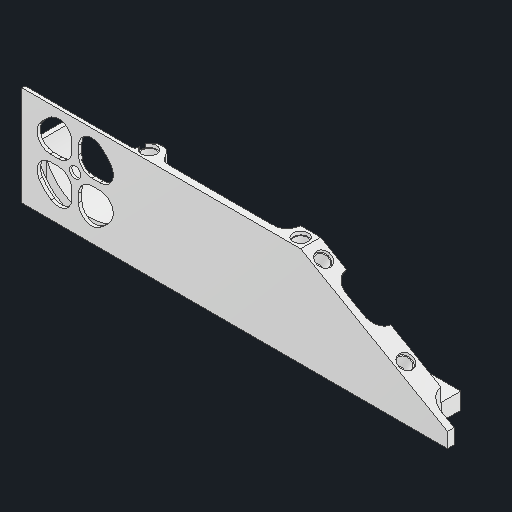
# Autodesk Inventor part: right_side
Saved by Autodesk Inventor 2023 (Build 270158000, 158)
## iProperties
Created: 2024-05-08
Part Number: right_side
Material: ABS Plastic
Document SubType Name: Modeling
Designer: szymo
Density: 1.06 g/cm^3
Appearance: Smooth - White
Mass: 9.52258 g
Surface Area: 89.3308 cm^2
Volume: 8.98357 cm^3
Author: szymo
Autodesk Inventor part; units mm, degrees
ref_plane "YZ Plane" through (0, 0, 0) normal (1, 0, 0) x (0, 1, 0)
ref_plane "XZ Plane" through (0, 0, 0) normal (0, 1, 0) x (-1, 0, 0)
ref_plane "XY Plane" through (0, 0, 0) normal (0, 0, 1) x (1, 0, 0)
sketch "Sketch1" plane through (0, 0, 0) normal (0, 0, 1) x (1, 0, 0)
  line L0 (128, 8) -> (128, 3.5) projected
  line L1 (128, 3.5) -> (132, 3.5) projected
  line L2 (132, 3.5) -> (132, 0) projected
  line L3 (132, 0) -> (146, 0) projected
  line L4 (146, 0) -> (132, 9) projected
  line L5 (132, 9) -> (132, 8) projected
  line L6 (132, 8) -> (128, 8) projected
  circle A0 centre (-25, 12) radius 22.5 projected
  line L7 (116.5, 3.5) -> (116.5, 11.1395) projected
  line L8 (116.5, 14.6395) -> (116.5, 11.1395) projected
  line L9 (109.1155, 18.903) -> (116.5, 14.6395)
  line L10 (109.1155, 18.903) -> (83.8327, 33.5)
  line L11 (47.75, 33.5) -> (83.8327, 33.5) projected
  line L12 (0, 3.5) -> (0, 31) projected
  line L13 (0, 3.5) -> (0, 33.5)
  line L14 (0, 33.5) -> (83.8327, 33.5)
  line L15 (83.8327, 33.5) -> (128, 8)
  line L16 (128, 3.5) -> (0, 3.5)
  point P0 (0, 0)
  constraints: 12 end point, 2 collinear, 1 parallel, 1 point on line
extrude "Extrusion1" add sketch "Sketch1" against normal blind 2 contours L0 L16 L7 L8 L15 | L8 L7 L16 L12 L13 L14 L11 L10 L9
sketch "Sketch2" plane through (0, 0, -2) normal (0, 0, -1) x (-1, 0, 0)
  circle A0 centre (-16, 19.5) radius 14 projected
  line L0 (0, 33.5) -> (-83.8327, 33.5) projected
  line L1 (-128, 3.5) -> (0, 3.5) projected
  line L2 (-33, 33.5) -> (0, 33.5)
  line L3 (0, 33.5) -> (0, 3.5)
  line L4 (0, 3.5) -> (-33, 3.5)
  line L5 (-33, 3.5) -> (-33, 33.5)
  point P0 (0, 0)
  point P1 (-116.5, 3.5)
  point P2 (-33, 3.5)
  dimension "d2" = 28
  dimension "d3" = 17
  constraints: 8 end point, 2 parallel, 1 horizontal, 1 perpendicular, 1 point on line
  measures "d2" diameter of A0
  measures "d3" distance from line of L5 A0.centre
extrude "Extrusion2" cut sketch "Sketch2" against normal blind 1 contours A0 | L0 L3 L1 L5
sketch "Sketch3" plane through (0, 0, -1) normal (0, 0, -1) x (-1, 0, 0)
  circle A0 centre (-16, 19.5) radius 14 projected
  line L0 (-33, 33.5) -> (0, 33.5) projected
  line L1 (-33, 3.5) -> (-33, 33.5) projected
  line L2 (0, 3.5) -> (-33, 3.5) projected
  line L3 (0, 33.5) -> (0, 3.5) projected
  line L4 (0, 3.5) -> (-128, 3.5) projected
  line L5 (0, 3.5) -> (-5, 3.5)
  line L6 (-5, 3.5) -> (-5, 6.5)
  line L7 (-5, 6.5) -> (0, 6.5)
  line L8 (0, 6.5) -> (0, 3.5)
  line L9 (-33, 3.5) -> (-28, 3.5)
  line L10 (-28, 3.5) -> (-28, 6.5)
  line L11 (-28, 6.5) -> (-33, 6.5)
  line L12 (-33, 6.5) -> (-33, 3.5)
  line L13 (-33, 9.5) -> (-25.798, 9.5)
  line L14 (-2.0052, 19.1168) -> (0, 18.5)
  line L15 (0, 33.5) -> (0, 3.5) projected
  point P0 (0, 0)
  point P1 (-116.5, 3.5)
  point P2 (0, 18.5)
  dimension "d6" = 5
  dimension "d7" = 3
  dimension "d8" = 5
  dimension "d9" = 3
  dimension "d10" = 3
  constraints: 20 end point, 4 parallel, 3 perpendicular, 3 point on line, 2 horizontal, 2 point on circle, 1 midpoint
  measures "d6" distance of L6.end L7.end
  measures "d7" distance of L5.end L6.end
  measures "d8" distance of L11.end L10.end
  measures "d9" distance of L10.end L9.end
  measures "d10" distance between parallel lines of L13 L11
ref_plane "Work Plane1" through (1, 4.5, -18.6) normal (0, 0, 1) x (1, 0, 0)
ref_plane "Work Plane2" through (1.675, 5.175, -4.8) normal (0, 0, 1) x (1, 0, 0)
extrude "Extrusion3" add sketch "Sketch3" along normal blind 6.8 contours A0 L14 L3 L7 L6 L2 L10 L11 L1 L13 | L11 L10 L2 L1 | L3 L2 L6 L7
sketch "Sketch4" plane through (0, 0, -7.8) normal (0, 0, -1) x (-1, 0, 0)
  circle A0 centre (-16, 19.5) radius 14 projected
  line L0 (-2.0052, 19.1168) -> (0, 18.5) projected
  line L1 (0, 33.5) -> (0, 18.5) projected
  line L2 (-33, 33.5) -> (0, 33.5) projected
  line L3 (-33, 9.5) -> (-33, 33.5) projected
  line L4 (-33, 9.5) -> (-25.798, 9.5) projected
  arc A1 (-25.798, 9.5) -> (-2.0052, 19.1168) centre (-16, 19.5) ccw projected
  line L5 (-29.9991, 19.6621) -> (-33, 19.6621)
  line L6 (-33, 9.5) -> (-33, 33.5) projected
  line L7 (0, 18.5) -> (-2.0052, 19.1168) projected
  line L8 (-2.0052, 19.1168) -> (0, 18.5)
  arc A2 (-25.798, 9.5) -> (-2.0052, 19.1168) centre (-16, 19.5) ccw projected
  line L9 (-25.798, 9.5) -> (-33, 9.5) projected
  line L10 (-33, 9.5) -> (-33, 3.5) projected
  line L11 (-33, 3.5) -> (0, 3.5) projected
  line L12 (0, 3.5) -> (0, 18.5) projected
  line L13 (0, 18.5) -> (-2.0052, 19.1168) projected
  point P0 (0, 0)
  constraints: 4 end point, 1 collinear, 1 perpendicular, 1 point on line, 2 other
ref_plane "Work Plane3" through (1, 4.5, -18.6) normal (0, 0, 1) x (1, 0, 0)
extrude "Extrusion4" add sketch "Sketch4" along normal blind 5 contours A0 L4 L3 L5 | A0 L0 L12 L11 L10 L4
sketch "Sketch5" plane through (25.798, 9.5, -1) normal (0, 1, 0) x (1, 0, 0)
  line L0 (7.202, 0) -> (0, 0) projected
  line L1 (7.202, 1) -> (7.202, 0) projected
  line L2 (7.202, 1) -> (7.202, 6.8) projected
  line L3 (0, 6.8) -> (7.202, 6.8) projected
  line L4 (0, 0) -> (0, 6.8) projected
  line L5 (7.202, 0) -> (0, 6.8)
  line L6 (0.7816, 0) -> (7.202, 6.8)
  point P0 (-25.798, -1)
  point P1 (3.9918, 3.4)
  constraints: 4 end point, 1 midpoint, 1 perpendicular, 1 point on line
hole "Hole1" at (29.7898, 9.5, -4.4) direction (0, -1, 0) diameter 3.6 end through all countersink diameter 6.5 countersink angle 90 clearance for "Countersunk Flat Head Screw ISO 2009/7046" size "M3" standard "ISO"
ref_plane "Work Plane4" through (41, 3.5, -89) normal (0, 1, 0) x (-1, 0, 0)
sketch "Sketch6" plane through (41, 3.5, -89) normal (0, 1, 0) x (-1, 0, 0)
  line L0 (8, 87) -> (-42.8327, 87) projected
  line L1 (-42.8327, 87) -> (-87, 87) projected
  line L2 (-87, 87) -> (8, 87) projected
  line L3 (-71, 89) -> (-71, 74) projected
  line L4 (-71, 74) -> (-87, 74) projected
  line L5 (-71, 87) -> (-64, 87)
  line L6 (-64, 87) -> (-64, 77)
  line L7 (-64, 77) -> (-71, 77)
  line L8 (-71, 77) -> (-71, 87)
  point P0 (41, 89)
  point P1 (-64, 87)
  dimension "d22" = 7
  dimension "d23" = 10
  constraints: 8 end point, 2 parallel, 2 point on line, 1 horizontal, 1 perpendicular
  measures "d22" distance of L6.end L7.end
  measures "d23" distance of L5.end L6.end
extrude "Extrusion5" add sketch "Sketch6" along normal blind 5
sketch "Sketch7" plane through (0, 0, -2) normal (0, 0, -1) x (-1, 0, 0)
  line L0 (-105, 8.5) -> (-105, 3.5) projected
  line L1 (-105, 3.5) -> (-33, 3.5) projected
  line L2 (-33, 3.5) -> (-33, 9.5) projected
  line L3 (-33, 9.5) -> (-33, 33.5) projected
  line L4 (-33, 33.5) -> (-83.8327, 33.5) projected
  line L5 (-83.8327, 33.5) -> (-128, 8) projected
  line L6 (-128, 8) -> (-128, 3.5) projected
  line L7 (-128, 3.5) -> (-112, 3.5) projected
  line L8 (-112, 3.5) -> (-112, 8.5) projected
  line L9 (-112, 8.5) -> (-105, 8.5) projected
  line L10 (-118.25, 3.5) -> (-115.75, 3.5) projected
  line L11 (-115.75, 3.5) -> (-118.25, 3.5)
  line L12 (-118.25, 3.5) -> (-118.25, 8.5)
  line L13 (-118.25, 8.5) -> (-115.75, 8.5)
  line L14 (-115.75, 8.5) -> (-115.75, 3.5)
  line L15 (-114, 3.5) -> (-120, 3.5)
  line L16 (-120, 3.5) -> (-120, 8.5)
  line L17 (-120, 8.5) -> (-114, 8.5)
  line L18 (-114, 8.5) -> (-114, 3.5)
  line L19 (-112, 8.5) -> (-114, 8.5)
  point P0 (0, 0)
  dimension "d26" = 5
  dimension "d27" = 6
  dimension "d28" = 1.75
  dimension "d29" = 1.75
  constraints: 18 end point, 4 parallel, 2 coincident, 2 horizontal, 2 perpendicular, 2 point on line, 1 collinear
  measures "d26" distance of L11.end L12.end
  measures "d27" distance of L16.end L17.end
  measures "d28" distance between parallel lines of L16 L12
  measures "d29" distance between parallel lines of L14 L18
extrude "Extrusion6" add sketch "Sketch7" along normal blind 10 contours L8 L7 L18 L19 | L18 L7 L14 L17 | L14 L7 L12 L13 | L12 L7 L16 L17
sketch "Sketch8" plane through (41, 8.5, -89) normal (0, 1, 0) x (1, 0, 0)
  line L0 (64, -77) -> (64, -87) projected
  line L1 (79, -87) -> (64, -87) projected
  line L2 (79, -87) -> (79, -77) projected
  line L3 (64, -77) -> (79, -77) projected
  line L4 (71, -77) -> (64, -83)
  line L5 (71, -89) -> (71, -74) projected
  point P0 (-41, -89)
  point P1 (67.5, -80)
  dimension "d40" = 4
  constraints: 3 point on line, 2 end point, 1 midpoint
  measures "d40" distance from line of L1 L4.end
hole "Hole2" at (108.5, 8.5, -9) direction (0, -1, 0) diameter 3.6 end through all countersink diameter 6 countersink angle 90 clearance for "Countersunk Flat Head Screw ISO 2009/7046" size "M3" standard "ISO"
sketch "Sketch9" plane through (0, 0, -2) normal (0, 0, -1) x (-1, 0, 0)
  line L0 (-120, 3.5) -> (-120, 8.5) projected
  line L1 (-120, 8.5) -> (-105, 8.5) projected
  line L2 (-105, 8.5) -> (-105, 3.5) projected
  line L3 (-105, 3.5) -> (-33, 3.5) projected
  line L4 (-33, 3.5) -> (-33, 9.5) projected
  line L5 (-33, 9.5) -> (-33, 33.5) projected
  line L6 (-33, 33.5) -> (-83.8327, 33.5) projected
  line L7 (-83.8327, 33.5) -> (-128, 8) projected
  line L8 (-128, 8) -> (-128, 3.5) projected
  line L9 (-128, 3.5) -> (-120, 3.5) projected
  line L10 (-105, 8.5) -> (-105, 21.2791)
  line L11 (0, 3.5) -> (-128, 3.5) projected
  line L12 (-128, 3.5) -> (-120, 3.5)
  line L13 (-120, 5.1132) -> (-120, 3.5)
  line L14 (-120, 5.1132) -> (-120, 8.5)
  line L15 (-120, 8.5) -> (-105, 8.5)
  line L16 (-122, 3.5) -> (-122, 11.4641)
  line L17 (-122, 3.5) -> (-114.0359, 3.5) construction
  line L18 (-33, 33.5) -> (0, 33.5) projected
  line L19 (-120, 8.5) -> (-120, 12.6188)
  line L20 (-128, 8) -> (-83.8327, 33.5) projected
  line L21 (-83.8327, 33.5) -> (-77.8327, 33.5)
  line L22 (-77.8327, 33.5) -> (-77.8327, 27.5)
  line L23 (-77.8327, 27.5) -> (-83.8327, 27.5)
  line L24 (-83.8327, 27.5) -> (-83.8327, 33.5)
  line L25 (-86.4308, 32) -> (-91.6269, 29)
  line L26 (-91.6269, 29) -> (-88.6269, 23.8038)
  line L27 (-88.6269, 23.8038) -> (-83.4308, 26.8038)
  line L28 (-83.4308, 26.8038) -> (-86.4308, 32)
  arc A0 (-77.8327, 27.5) -> (-88.6269, 23.8038) centre (-78.8572, 12.8822) ccw
  point P0 (0, 0)
  point P1 (-128, 5.75)
  dimension "d41" = 90
  dimension "d42" = 6
  dimension "d139" = 6
  dimension "d140" = 6
  dimension "d141" = 6
  dimension "d142" = 6
  constraints: 32 end point, 8 point on line, 4 collinear, 4 parallel, 3 perpendicular, 3 point on circle, 2 horizontal, 2 vertical, 1 centre point, 1 midpoint
  measures "d41" angle of L17 L16
  measures "d42" distance from line of L16 point (-128, 5.75)
  measures "d139" distance of L22.end L23.end
  measures "d140" distance of L21.end L22.end
  measures "d141" distance of L25.start L25.end
  measures "d142" distance of L26.end L25.end
extrude "zeberka" add sketch "Sketch9" along normal blind 4 contours L19 L7 L10 L1 | L7 L28 A0 L26 | L7 L24 L28 | L22 A0 L23 L24 L6 | L23 A0 L28
sketch "Sketch11" plane through (0, 0, -2) normal (0, 0, -1) x (-1, 0, 0)
  line L0 (-33, 9.5) -> (-33, 33.5) projected
  line L1 (-33, 33.5) -> (-39, 33.5)
  line L2 (-39, 33.5) -> (-39, 27.5)
  line L3 (-39, 27.5) -> (-33, 27.5)
  line L4 (-33, 27.5) -> (-33, 33.5)
  point P0 (0, 0)
  dimension "d63" = 6
  dimension "d64" = 6
  constraints: 8 end point, 2 parallel, 1 horizontal, 1 perpendicular
  measures "d63" distance of L3.end L2.end
  measures "d64" distance of L2.end L1.end
extrude "Extrusion8" add sketch "Sketch11" along normal blind 4
fillet "Fillet1" radius 3 3 edges at (39, 30.5, -2) (39, 30.5, -6) (33, 30.5, -6)
chamfer "Chamfer1" distance 4 angle 45 2 edges at (40.5, 27.5, -2) (36, 27.5, -2)
sketch "Sketch18" plane through (0, 0, 0) normal (0, 0, 1) x (1, 0, 0)
  circle A0 centre (16, 19.5) radius 14 projected
  circle A1 centre (16, 19.5) radius 5 projected
  circle A2 centre (16, 19.5) radius 13
  line L0 (15, 33.5) -> (17, 33.5)
  line L1 (17, 33.5) -> (17, 5.5)
  line L2 (17, 5.5) -> (15, 5.5)
  line L3 (15, 5.5) -> (15, 33.5)
  line L4 (2.0358, 20.5) -> (30, 20.5)
  line L5 (30, 20.5) -> (30, 18.5)
  line L6 (30, 18.5) -> (2.0358, 18.5)
  line L7 (2.0358, 18.5) -> (2.0358, 20.5)
  arc A3 (11.101, 20.5) -> (15, 24.399) centre (11.0012, 24.4988) ccw
  arc A4 (17, 24.399) -> (20.899, 20.5) centre (20.9988, 24.4988) ccw
  arc A5 (20.899, 18.5) -> (17, 14.601) centre (20.9988, 14.5012) ccw
  arc A6 (15, 14.601) -> (11.101, 18.5) centre (11.0012, 14.5012) ccw
  point P0 (0, 0)
  point P1 (15, 13.9299)
  point P2 (11.5241, 17.875)
  point P3 (3.0385, 18.5)
  point P4 (15, 6.5385)
  point P5 (17, 6.5385)
  point P6 (28.9615, 18.5)
  point P7 (19.5854, 18.5)
  point P8 (16.2425, 14.6027)
  point P9 (16.2425, 24.3973)
  point P10 (19.5854, 20.5)
  point P11 (28.9615, 20.5)
  point P12 (17, 32.4615)
  point P13 (11.4499, 20.5)
  point P14 (14.375, 23.4753)
  point P15 (15, 32.4615)
  point P16 (3.0385, 20.5)
  point P17 (15, 20.5)
  point P18 (17, 20.5)
  point P19 (15, 18.5)
  point P20 (17, 18.5)
  point P21 (29.9642, 18.5)
  point P22 (30, 19.5)
  point P23 (29.9642, 20.5)
  point P24 (15, 5.5358)
  point P25 (16, 5.5)
  point P26 (17, 5.5358)
  dimension "d104" = 1
  dimension "d111" = 1
  dimension "d112" = 1
  dimension "d113" = 1
  dimension "d114" = 1
  dimension "d115" = 4
  dimension "d116" = 4
  dimension "d117" = 4
  dimension "d118" = 4
  constraints: 16 end point, 8 point on circle, 8 point on line, 5 centre point, 4 horizontal, 4 parallel, 2 perpendicular, 1 vertical, 11 other
  measures "d111" distance from line of A2.centre L1
  measures "d112" distance from line of L3 A2.centre
  measures "d113" distance from line of L4 A2.centre
  measures "d114" distance from line of point (16, 19.5) L6
  measures "d115" radius of A3
  measures "d116" radius of A4
  measures "d117" radius of A5
  measures "d118" radius of A6
extrude "Extrusion11" cut sketch "Sketch18" against normal up to next contours A2 L3 A1 L4 | L6 A1 L3 A2 | A3 L3 L4 | A1 A3 | A6 A1 | L6 L3 A6 | A2 L4 A1 L1 | L1 A1 L6 A2 | A4 L4 L1 | A1 A4 | A5 A1 | L1 L6 A5
fillet "Fillet2" radius 4 12 edges at (3.0385, 20.5, -0.5) (3.0385, 18.5, -0.5) (15, 6.5385, -0.5) (17, 6.5385, -0.5) (28.9615, 18.5, -0.5) (28.9615, 20.5, -0.5) (17, 32.4615, -0.5) (15, 32.4615, -0.5) (17, 20.5, -0.5) (17, 18.5, -0.5) (15, 18.5, -0.5) (15, 20.5, -0.5)
sketch "Sketch19" plane through (0, 3.5, -12.8) normal (0, -1, 0) x (1, 0, 0)
  line L0 (2, 8.4) -> (30, 8.4) projected
  line L1 (2, 8.4) -> (25.798, 8.4)
  line L2 (25.798, 8.4) -> (25.798, 10.4)
  line L3 (25.798, 10.4) -> (2, 10.4)
  line L4 (2, 10.4) -> (2, 8.4)
  line L5 (25.798, 11.8) -> (25.798, 5) projected
  point P0 (0, 12.8)
  dimension "d122" = 2
  constraints: 8 end point, 2 parallel, 1 collinear, 1 horizontal, 1 perpendicular
  measures "d122" distance of L2.end L1.end
extrude "Extrusion12" cut sketch "Sketch19" against normal up to next
sketch "Sketch20" plane through (0, 3.5, -12.8) normal (0, -1, 0) x (1, 0, 0)
  circle A0 centre (117, 3.8) radius 1.25 projected
  point P0 (0, 12.8)
  constraints: 1 coincident
hole "Hole6" at (117, 3.5, -9) direction (0, 1, 0) diameter 3 depth 4 counterbore diameter 3.5 counterbore depth 1
fillet "Fillet5" radius 2 2 edges at (33, 19.6621, -10.3) (29.9991, 19.6621, -10.3)
fillet "Fillet6" radius 1 4 edges at (25.798, 6.5, -2.4) (2, 11.3076, -2.4) (2, 11.3076, -4.4) (25.798, 6.5, -4.4)
fillet "Fillet7" radius 1 1 edges at (33, 21.5, -1)
fillet "Fillet9" radius 4.25 6 edges at (77.8327, 27.5, -4) (88.6269, 23.8038, -4) (90.1269, 26.4019, -2) (77.8327, 30.5, -2) (105, 12.3895, -2) (120, 8.0594, -2)
chamfer "Chamfer2" distance 4 angle 45 1 edges at (83.3894, 26.8174, -2)
sketch "Sketch21" plane through (0, 33.5, 0) normal (0, 1, 0) x (1, 0, 0)
  arc A0 (39.1716, 4) -> (36.3431, 6) centre (36.3431, 3) ccw projected
  line L0 (36, 6) -> (36.3431, 6) projected
  arc A1 (36, 6) -> (33, 3) centre (36, 3) ccw projected
  line L1 (33, 3) -> (33, 2) projected
  arc A2 (32, 1) -> (33, 2) centre (32, 2) ccw projected
  line L2 (32, 1) -> (0, 1) projected
  line L3 (0, 0) -> (0, 1) projected
  line L4 (83.8327, 0) -> (0, 0) projected
  line L5 (83.8327, 0) -> (83.8327, 6) projected
  line L6 (77.8327, 6) -> (83.8327, 6) projected
  arc A3 (73.5901, 2) -> (77.8327, 6) centre (73.5901, 6.25) ccw projected
  line L7 (42, 2) -> (73.5901, 2) projected
  arc A4 (39.1716, 4) -> (42, 2) centre (42, 5) ccw projected
  line L8 (77.8327, 6) -> (83.8327, 0)
  point P0 (0, 0)
  point P1 (35.2466, 3)
  point P2 (80.8327, 3)
  constraints: 2 end point, 1 midpoint
hole "Hole7" at (35.2466, 33.5, -3) at (80.8327, 33.5, -3) direction (0, -1, 0) diameter 4 depth 5 counterbore diameter 4.6 counterbore depth 1
sketch "Sketch22" plane through (128, 8, 0) normal (0.5, 0.8660254, 0) x (0.8660254, -0.5, 0)
  line L0 (0, 0) -> (-51, 0) projected
  line L1 (0, 0) -> (0, 2) projected
  line L2 (-4.3301, 2) -> (0, 2) projected
  ellipse E0 centre (-4.3301, 6.25) end of major axis (0.5774, 6.25) minor radius 4.25 (-9.2291, 6) -> (-4.3301, 2) ccw projected
  line L3 (-26.5666, 6) -> (-9.2291, 6) projected
  ellipse E1 centre (-31.4656, 6.25) end of major axis (-26.5581, 6.25) minor radius 4.25 (-31.4656, 2) -> (-26.5666, 6) ccw projected
  line L4 (-37.7574, 2) -> (-31.4656, 2) projected
  arc A0 (-42, 6) -> (-37.7574, 2) centre (-37.7574, 6.25) ccw projected
  line L5 (-51, 6) -> (-42, 6) projected
  line L6 (-51, 0) -> (-51, 6) projected
  line L7 (-42, 6) -> (-51, 0)
  line L8 (-17.8979, 0) -> (-17.8979, 6)
  point P0 (-106.8513, 0)
  point P1 (-17.8979, 3)
  point P2 (-46.5, 3)
  dimension "d154" = 8.6687
  dimension "d155" = 8.6687
  constraints: 4 end point, 3 midpoint, 1 perpendicular, 1 point on line, 2 other
  measures "d154" distance from line of L8 L3.start
  measures "d155" distance of L3.end L8.end
hole "Hole8" at (112.5, 16.9489, -3) at (87.7298, 31.25, -3) direction (-0.5, -0.8660254, 0) diameter 4 depth 5 counterbore diameter 4.6 counterbore depth 1
sketch "Sketch23" plane through (0, 0, -1) normal (0, 0, -1) x (-1, 0, 0)
  circle A0 centre (-16, 19.5) radius 3.25
  circle A1 centre (-16, 19.5) radius 3.75
  point P0 (0, 0)
  dimension "d167" = 0.5
  constraints: 2 centre point, 2 other
  measures "d167" radial gap between concentric circles of A0 A1
ref_plane "Work Plane5" through (12.75, 16.25, -0.7) normal (0, 0, 1) x (1, 0, 0)
extrude "Extrusion13" cut sketch "Sketch23" against normal up to surface (0.3 mm away) contours A0 | A1
sketch "Sketch24" plane through (16, 19.5, 0) normal (0, 0, -1) x (-1, 0, 0)
  circle A0 centre (0, 0) radius 1.2
  circle A1 centre (0, 0) radius 3.25
  circle A2 centre (0, 0) radius 1.7
  point P0 (16, -19.5)
  dimension "d168" = 0.5
  constraints: 3 centre point, 4 other
  measures "d168" radial gap between concentric circles of A0 A2
extrude "Extrusion14" cut sketch "Sketch24" along normal up to next contours A0 | A2
equation "\"d28\" = d29"
body "Solid1"
